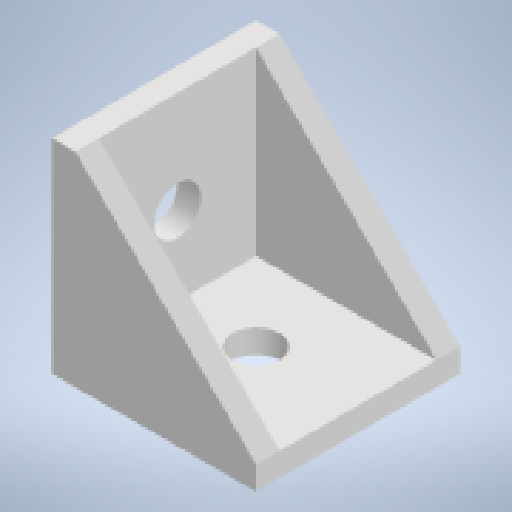
# Autodesk Inventor part: Escuadra
Saved by Autodesk Inventor 2023 (Build 270158000, 158)
## iProperties
Created: 2022-12-03
Part Number: Escuadra
Material: Genérico
Document SubType Name: Modeling
Designer: sergi
Density: 1 g/cm^3
Appearance: Valor por defecto
Author: sergi
Autodesk Inventor part; units mm, degrees
ref_plane "YZ Plane" through (0, 0, 0) normal (1, 0, 0) x (0, 1, 0)
ref_plane "XZ Plane" through (0, 0, 0) normal (0, 1, 0) x (-1, 0, 0)
ref_plane "XY Plane" through (0, 0, 0) normal (0, 0, 1) x (1, 0, 0)
sketch "Boceto1" plane through (0, 0, 0) normal (0, 1, 0) x (-1, 0, 0)
  line L0 (-6.5, -6.5) -> (6.5, -6.5)
  line L1 (6.5, -6.5) -> (6.5, 6.5)
  line L2 (6.5, 6.5) -> (-6.5, 6.5)
  line L3 (-6.5, 6.5) -> (-6.5, -6.5)
  line L4 (-6.5, -6.5) -> (6.5, 6.5) construction
  line L5 (6.5, -6.5) -> (-6.5, 6.5) construction
  point P0 (0, 0)
  dimension "d0" = 13
  dimension "d1" = 13
  constraints: 12 end point, 2 midpoint, 2 parallel, 1 horizontal, 1 perpendicular
  measures "d0" distance of L2.end L1.end
  measures "d1" distance of L1.end L0.end
extrude "Extrusión1" add sketch "Boceto1" along normal blind 13
shell "Vaciado1" thickness 1.5 removed faces 2 at (6.5, 4.3333, 2.1667) at (-2.1667, 13, -2.1667)
chamfer "Chaflán1" distance 11.5 angle 45 2 edges at (6.5, 13, 5.75) (6.5, 13, -5.75)
sketch "Boceto2" plane through (0, 0, 0) normal (0, -1, 0) x (1, 0, 0)
  line L0 (-6.5, 6.5) -> (6.5, 6.5) projected
  line L1 (-6.5, -6.5) -> (-6.5, 6.5) projected
  point P0 (0, 0)
  point P1 (0, 0)
  dimension "d8" = 6.5
  dimension "d9" = 6.5
  measures "d8" distance from line of L0 point (0, 0)
  measures "d9" distance from line of L1 point (0, 0)
hole "Agujero1" at (0, 0, 0) direction (0, 1, 0) diameter 3 depth 3 tip angle 118
sketch "Boceto3" plane through (-6.5, 0, -6.5) normal (-1, 0, 0) x (0, 0, 1)
  line L0 (0, 0) -> (13, 0) projected
  line L1 (13, 0) -> (13, 13) projected
  point P0 (6.5, 0)
  point P1 (6.5, 6.5)
  dimension "d17" = 6.5
  dimension "d18" = 6.5
  measures "d17" distance from line of L0 point (6.5, 6.5)
  measures "d18" distance from line of L1 point (6.5, 6.5)
hole "Agujero2" at (-6.5, 6.5, 0) direction (1, 0, 0) diameter 3 depth 3 tip angle 118
